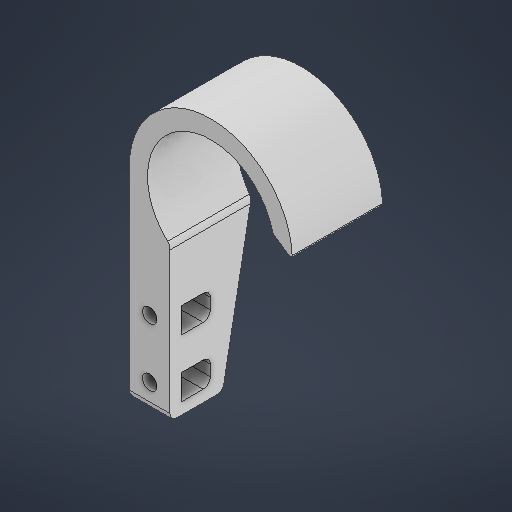
# Autodesk Inventor part: крюк старый
Saved by Autodesk Inventor 2025 (Build 290162000, 162)
## iProperties
Created: 2024-12-14
Part Number: крюк старый
Material: Типовые
Document SubType Name: Modeling
Designer: Phantom
Density: 1 g/cm^3
Appearance: По умолчанию
Author: Phantom
Autodesk Inventor part; units mm, degrees
ref_plane "YZ Plane" through (0, 0, 0) normal (1, 0, 0) x (0, 1, 0)
ref_plane "XZ Plane" through (0, 0, 0) normal (0, 1, 0) x (-1, 0, 0)
ref_plane "XY Plane" through (0, 0, 0) normal (0, 0, 1) x (1, 0, 0)
sketch "Эскиз1" plane through (0, 0, 0) normal (0, 0, 1) x (1, 0, 0)
  arc A0 (16.937, 4.4032) -> (-11.9308, -12.8026) centre (0, 0) ccw
  arc A1 (22.4785, 0.9844) -> (-22.5, 0) centre (0, 0) ccw
  line L0 (-22.5, 0) -> (-22.5, -55)
  line L1 (-22.5, 0) -> (32.5, 0) construction
  line L2 (-22.5, -55) -> (-17.5, -55)
  line L3 (21.6965, 0.5499) -> (17.743, 3.256)
  arc A2 (-11.3173, -14.5681) -> (-11.9308, -12.8026) centre (-13.2943, -14.2658) ccw
  arc A3 (16.937, 4.4032) -> (17.743, 3.256) centre (18.8727, 4.9064) ccw
  arc A4 (21.6965, 0.5499) -> (22.4785, 0.9844) centre (21.9789, 0.9626) ccw
  line L4 (-11.3173, -14.5681) -> (-11.3173, -55)
  line L5 (-11.3173, -55) -> (-17.5, -55)
  point P0 (22.5, 0)
  point P1 (-11.1519, -13.4865)
  point P2 (17.1061, 3.6919)
  dimension "d0" = 35
  dimension "d1" = 45
  dimension "d2" = 55
  dimension "d3" = 90
  dimension "d4" = 5
  dimension "d5" = 2
  dimension "d6" = 0.5
  constraints: 13 point on circle, 12 end point, 5 centre point, 5 tangent, 3 perpendicular, 3 point on line, 2 coincident, 2 vertical, 1 equal radius, 1 horizontal
  measures "d0" diameter of A0
  measures "d1" diameter of A1
  measures "d2" distance of L0.start L0.end
  measures "d3" angle of L0 L1
  measures "d4" distance of L0.end L2.end
  measures "d5" radius of A2
  measures "d6" radius of A4
extrude "Выдавливание1" add sketch "Эскиз1" along normal blind 25
sketch "Эскиз2" plane through (0, 0, 25) normal (0, 0, 1) x (1, 0, 0)
  line L0 (-22.5, -55) -> (-11.3173, -55) projected
  line L1 (-16.9086, -55) -> (-16.9086, -49)
  circle A0 centre (-16.9086, -49) radius 2
  line L2 (-16.9086, -49) -> (-16.9086, -33)
  circle A1 centre (-16.9086, -33) radius 2
  point P0 (0, 0)
  dimension "d9" = 6
  dimension "d10" = 4
  dimension "d11" = 16
  dimension "d12" = 4
  constraints: 4 end point, 2 centre point, 2 coincident, 2 vertical, 1 midpoint
  measures "d9" distance of L1.start L1.end
  measures "d10" diameter of A0
  measures "d11" distance of L2.start L2.end
  measures "d12" diameter of A1
extrude "Выдавливание2" cut sketch "Эскиз2" against normal blind 10
sketch "Эскиз3" plane through (-22.5, -55, 0) normal (-1, 0, 0) x (0, 0, 1)
  line L0 (25, 24) -> (25, 20) projected
  line L1 (25, 8) -> (25, 4) projected
  line L2 (25, 20) -> (25, 18.5)
  line L3 (25, 8) -> (25, 11)
  line L4 (0, 55) -> (0, 0) projected
  line L5 (25, 18.5) -> (0, 18.5)
  line L6 (0, 18.5) -> (0, 9.5)
  line L7 (0, 9.5) -> (25, 9.5)
  line L8 (25, 9.5) -> (25, 18.5)
  line L9 (21.8, 18.5) -> (21.8, 9.5)
  line L10 (21.8, 18.5) -> (13.8, 18.5)
  line L11 (13.8, 18.5) -> (13.8, 9.5)
  line L12 (21.8, 9.5) -> (13.8, 9.5)
  line L13 (25, 24) -> (25, 25.5)
  line L14 (21.8, 18.5) -> (13.8, 18.5)
  line L15 (25, 24) -> (25, 4)
  line L16 (25, 14) -> (-3.5354, 14)
  line L17 (21.8, 9.5) -> (13.8, 9.5)
  line L18 (25, 4) -> (25, 2.5)
  line L19 (25, 20) -> (15, 20) projected
  line L20 (21.8, 20) -> (13.8, 20)
  line L21 (13.8, 20) -> (13.8, 25.5)
  line L22 (13.8, 25.5) -> (21.8, 25.5)
  line L23 (21.8, 25.5) -> (21.8, 20)
  line L24 (21.8, 8) -> (13.8, 8)
  line L25 (13.8, 8) -> (13.8, 2.5)
  line L26 (13.8, 2.5) -> (21.8, 2.5)
  line L27 (21.8, 2.5) -> (21.8, 8)
  line L28 (21.8, 18.5) -> (13.8, 18.5)
  line L29 (13.8, 18.5) -> (13.8, 20)
  line L30 (13.8, 20) -> (21.8, 20)
  line L31 (21.8, 20) -> (21.8, 18.5)
  line L32 (21.8, 8) -> (13.8, 8)
  line L33 (13.8, 8) -> (13.8, 9.5)
  line L34 (13.8, 9.5) -> (21.8, 9.5)
  line L35 (21.8, 9.5) -> (21.8, 8)
  point P0 (15, 8)
  point P1 (21.8, 9.5)
  point P2 (13.8, 9.5)
  dimension "d15" = 1.5
  dimension "d16" = 3
  dimension "d18" = 8
  dimension "d21" = 1.5
  constraints: 64 end point, 8 parallel, 7 perpendicular, 7 symmetric about line, 6 point on line, 5 horizontal, 2 collinear, 1 midpoint
  measures "d15" distance of L0.end L2.end
  measures "d16" distance of L1.start L3.end
  measures "d18" distance of L9.start L10.end
  measures "d21" distance of L0.start L13.end
extrude "Выдавливание3" cut sketch "Эскиз3" against normal through all contours L31 L5 L29 L20 L19 | L19 L20 L21 L22 L23 | L35 L24 L33 L7 | L27 L26 L25 L24
sketch "Эскиз4" plane through (-22.5, -55, 0) normal (0, -1, 0) x (1, 0, 0)
  line L0 (0, 0) -> (11.1827, 0) projected
  line L1 (11.1827, 0) -> (11.1827, 25) projected
  line L2 (0, 25) -> (11.1827, 25) projected
  line L3 (0, 0) -> (0, 25) projected
  point P0 (22.5, 0)
extrude "Выдавливание4" add sketch "Эскиз4" along normal blind 0.7
sketch "Эскиз5" plane through (-22.5, 0, 0) normal (-1, 0, 0) x (0, 0, 1)
  line L0 (13.8, -52.5) -> (21.8, -52.5) projected
  line L1 (0, 0) -> (0, -55.7) projected
  line L2 (9.8, -52.5) -> (0, 0)
  line L3 (25, -55.7) -> (0, -55.7) projected
  line L4 (9.8, -52.5) -> (10.3973, -55.7)
  dimension "d24" = 4
  constraints: 4 end point, 1 point on line
  measures "d24" distance of L0.start L2.start
extrude "Выдавливание5" cut sketch "Эскиз5" against normal through all
fillet "Сопряжение1" radius 2 4 edges at (-16.9086, -36.5, 13.8) (-16.9086, -29.5, 13.8) (-16.9086, -52.5, 13.8) (-16.9086, -45.5, 13.8)
fillet "Сопряжение2" radius 2 2 edges at (-16.9086, -55.7, 10.3973) (-16.9086, -55.7, 25)
